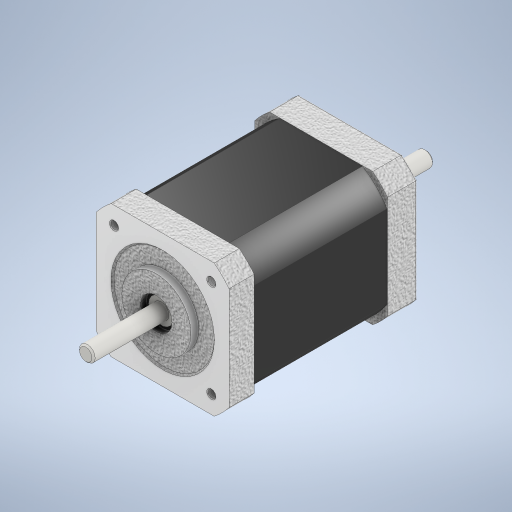
# Autodesk Inventor part: NEMA 17 Y-axis
Saved by Autodesk Inventor 2024 (Build 280153000, 153)
## iProperties
Created: 2021-02-07
Part Number: NEMA 17 Y-axis
Material: Aluminum 6061
Document SubType Name: Modeling
Designer: Ishaan
Density: 2.7 g/cm^3
Appearance: Aluminum Cast
Author: Ishaan
Autodesk Inventor part; units mm, degrees
sketch "Sketch1" plane through (0, 0, 0) normal (0, 0, 1) x (1, 0, 0)
  line L0 (21.15, -21.15) -> (-21.15, -21.15)
  line L1 (-21.15, -21.15) -> (-21.15, 21.15)
  line L2 (-21.15, 21.15) -> (21.15, 21.15)
  line L3 (21.15, 21.15) -> (21.15, -21.15)
  line L4 (21.15, -21.15) -> (-21.15, 21.15) construction
  line L5 (-21.15, -21.15) -> (21.15, 21.15) construction
  line L6 (15.5, -15.5) -> (-15.5, -15.5) construction
  line L7 (-15.5, -15.5) -> (-15.5, 15.5) construction
  line L8 (-15.5, 15.5) -> (15.5, 15.5) construction
  line L9 (15.5, 15.5) -> (15.5, -15.5) construction
  line L10 (15.5, -15.5) -> (-15.5, 15.5) construction
  line L11 (-15.5, -15.5) -> (15.5, 15.5) construction
  circle A0 centre (0, 0) radius 24.95
  circle A1 centre (0, 0) radius 11
  circle A2 centre (0, 0) radius 26.775
  point P0 (-13.2356, 21.15)
  point P1 (-21.15, 13.2356)
  point P2 (-21.15, -13.2356)
  point P3 (-13.2356, -21.15)
  point P4 (13.2356, -21.15)
  point P5 (21.15, -13.2356)
  point P6 (21.15, 13.2356)
  point P7 (13.2356, 21.15)
  point P8 (16.4188, -21.15)
  point P9 (21.15, -16.4188)
  point P10 (-21.15, -16.4188)
  point P11 (-16.4188, -21.15)
  point P12 (-16.4188, 21.15)
  point P13 (-21.15, 16.4188)
  point P14 (21.15, 16.4188)
  point P15 (16.4188, 21.15)
  dimension "d0" = 42.3
  dimension "d1" = 42.3
  dimension "d2" = 31
  dimension "d3" = 31
  dimension "d4" = 49.9
  dimension "d5" = 22
  dimension "d90" = 53.55
  constraints: 24 end point, 7 coincident, 4 midpoint, 4 parallel, 3 centre point, 2 horizontal, 2 perpendicular
  measures "d0" distance of L1.end L2.end
  measures "d1" distance of L0.end L1.end
  measures "d2" distance of L7.end L8.end
  measures "d3" distance of L6.end L7.end
  measures "d4" diameter of A0
  measures "d5" diameter of A1
  measures "d90" diameter of A2
extrude "Extrusion1" add sketch "Sketch1" against normal blind 8 contours L0 A0 L3 A2 | L0 A0 L1 L2 L3 | A2 L1 A0 L0 | A0 L2 A2 L3 | A2 L2 A0 L1 | A1
extrude "Extrusion2" add sketch "Sketch1" along normal blind 2 contours A1
hole "Hole1" at (-15.5, 15.5, 0) at (15.5, 15.5, 0) at (15.5, -15.5, 0) at (-15.5, -15.5, 0) direction (0, 0, -1) diameter 2.459 depth 4.5 thread size "M3x0.5" class "6H" standard "ANSI Metric M Profile"
ref_plane "Work Plane1" through (0, 0, -60) normal (0, 0, 1) x (1, 0, 0)
sketch "Sketch2" plane through (0, 0, -60) normal (0, 0, 1) x (1, 0, 0)
  line L0 (-16.4188, 21.15) -> (16.4188, 21.15) projected
  line L1 (21.15, 16.4188) -> (21.15, -16.4188) projected
  line L2 (16.4188, -21.15) -> (-16.4188, -21.15) projected
  line L3 (-21.15, -16.4188) -> (-21.15, 16.4188) projected
  arc A0 (-16.4188, 21.15) -> (-21.15, 16.4188) centre (0, 0) ccw projected
  arc A1 (21.15, 16.4188) -> (16.4188, 21.15) centre (0, 0) ccw projected
  arc A2 (16.4188, -21.15) -> (21.15, -16.4188) centre (0, 0) ccw projected
  arc A3 (-21.15, -16.4188) -> (-16.4188, -21.15) centre (0, 0) ccw projected
extrude "Extrusion3" add sketch "Sketch2" along normal blind 9.5
sketch "Sketch3" plane through (0, 0, -8) normal (0, 0, -1) x (-1, 0, 0)
  line L0 (16.4188, 21.15) -> (-16.4188, 21.15) projected
  line L1 (-21.15, 16.4188) -> (-21.15, -16.4188) projected
  line L2 (-16.4188, -21.15) -> (16.4188, -21.15) projected
  line L3 (21.15, -16.4188) -> (21.15, 16.4188) projected
  circle A0 centre (0, 0) radius 11 projected
  circle A1 centre (0, 0) radius 24.925
  line L4 (13.2068, -21.05) -> (-13.2068, -21.05)
  arc A2 (-21.05, -13.2068) -> (-13.2068, -21.05) centre (0, 0) ccw
  line L5 (-21.05, -13.2068) -> (-21.05, 13.2068)
  arc A3 (-13.2068, 21.05) -> (-21.05, 13.2068) centre (0, 0) ccw
  line L6 (-13.2068, 21.05) -> (13.2068, 21.05)
  arc A4 (21.05, 13.2068) -> (13.2068, 21.05) centre (0, 0) ccw
  line L7 (21.05, 13.2068) -> (21.05, -13.2068)
  arc A5 (13.2068, -21.05) -> (21.05, -13.2068) centre (0, 0) ccw
  arc A6 (21.15, 16.4188) -> (16.4188, 21.15) centre (0, 0) ccw projected
  arc A7 (-16.4188, 21.15) -> (-21.15, 16.4188) centre (0, 0) ccw projected
  arc A8 (-21.15, -16.4188) -> (-16.4188, -21.15) centre (0, 0) ccw projected
  arc A9 (16.4188, -21.15) -> (21.15, -16.4188) centre (0, 0) ccw projected
  point P0 (21.15, 13.1884)
  point P1 (13.1884, 21.15)
  point P2 (-13.1884, 21.15)
  point P3 (-21.15, 13.1884)
  point P4 (-21.15, -13.1884)
  point P5 (-13.1884, -21.15)
  point P6 (13.1884, -21.15)
  point P7 (21.15, -13.1884)
  point P8 (21.05, -13.7173)
  point P9 (21.05, 13.7173)
  point P10 (13.7173, 21.05)
  point P11 (-13.7173, 21.05)
  point P12 (-21.05, 13.7173)
  point P13 (-21.05, -13.7173)
  point P14 (-13.7173, -21.05)
  point P15 (13.7173, -21.05)
  dimension "d20" = 49.85
  dimension "d23" = 0.1
  constraints: 8 end point, 8 point on circle, 5 centre point, 1 coincident
  measures "d20" diameter of A1
  measures "d23" distance between parallel lines of L2 L4
extrude "Extrusion5" add sketch "Sketch3" along normal up to surface (42.5 mm away) contours L4 A2 L5 A3 L6 A4 L7 A5
chamfer "Chamfer1" distance 0.25 angle 45 4 edges at (-15.5, 16.7295, 0) (15.5, 16.7295, 0) (15.5, -14.2705, 0) (-15.5, -14.2705, 0)
sketch "Sketch4" plane through (0, 0, 2) normal (0, 0, 1) x (1, 0, 0)
  circle A0 centre (0, 0) radius 11 projected
  constraints: 1 coincident
hole "Hole2" at (0, 0, 2) direction (0, 0, -1) diameter 10 depth 2
sketch "Sketch5" plane through (0, 0, 0) normal (0, 0, 1) x (1, 0, 0)
  circle A0 centre (0, 0) radius 2.5
  circle A1 centre (0, 0) radius 4
  line L0 (-1.5, -2) -> (1.5, -2)
  dimension "d36" = 5
  dimension "d37" = 8
  dimension "d41" = 4.5
  constraints: 2 centre point, 2 coincident, 2 end point, 2 point on circle, 1 horizontal
  measures "d36" diameter of A0
  measures "d37" diameter of A1
ref_plane "Work Plane2" through (0, 0, 24.5) normal (0, 0, 1) x (1, 0, 0)
extrude "Extrusion6" add sketch "Sketch5" along normal up to surface (24.5 mm away) contours A0 L0 | L0 A0
chamfer "Chamfer2" distance 0.5 angle 45 1 edges at (1.5, 2, 24.5)
extrude "Extrusion7" cut sketch "Sketch5" along normal blind 22.298 from surface at 2 contours L0 A0 picked at (-0.3466, -2.0912)
extrude "Extrusion8" add sketch "Sketch5" along normal blind 0.5
sketch "Sketch6" plane through (0, 0, -60) normal (0, 0, -1) x (-1, 0, 0)
  circle A0 centre (0, 0) radius 5
  dimension "d49" = 10
  constraints: 1 centre point, 1 coincident
  measures "d49" diameter of A0
extrude "Extrusion9" cut sketch "Sketch6" against normal blind 3
sketch "Sketch7" plane through (0, 0, -57) normal (0, 0, -1) x (-1, 0, 0)
  circle A0 centre (0, 0) radius 4
  circle A1 centre (0, 0) radius 2.5
  dimension "d52" = 8
  dimension "d53" = 5
  constraints: 2 centre point, 2 coincident
  measures "d52" diameter of A0
  measures "d53" diameter of A1
ref_plane "Work Plane4" through (0, 0, -84) normal (0, 0, -1) x (-1, 0, 0)
extrude "Extrusion10" add sketch "Sketch7" along normal up to surface (27 mm away) contours A1
ref_plane "Work Plane5" through (0, 0, -69) normal (0, 0, -1) x (-1, 0, 0)
chamfer "Chamfer5" distance 0.5 angle 45 1 edges at (2.5, 0, -84)
sketch "Sketch11" plane through (0, 0, -69) normal (0, 0, -1) x (-1, 0, 0)
  circle A0 centre (0, 0) radius 2.5 projected
  line L0 (1.5, -2) -> (-1.5, -2)
  dimension "d94" = 2
  constraints: 2 end point, 2 point on circle, 1 horizontal
  measures "d94" distance from line of L0 point (0, 0)
extrude "Extrusion15" cut sketch "Sketch11" along normal through all contours L0 A0 picked at (-0.3466, -2.0912)
extrude "Extrusion11" add sketch "Sketch7" along normal blind 0.5
sketch "Sketch8" plane through (0, 0, -60) normal (0, 0, -1) x (-1, 0, 0)
  circle A0 centre (-15.5, 15.5) radius 1.2295 projected
  circle A1 centre (-15.5, 15.5) radius 3.25
  circle A2 centre (15.5, 15.5) radius 1.2295 projected
  circle A3 centre (15.5, 15.5) radius 3.25
  circle A4 centre (15.5, -15.5) radius 3.25
  circle A5 centre (-15.5, -15.5) radius 1.2295 projected
  circle A6 centre (-15.5, -15.5) radius 3.25
  line L0 (12.25, -21.15) -> (-12.25, -21.15)
  line L1 (-12.25, -21.15) -> (-12.25, 21.15)
  line L2 (-12.25, 21.15) -> (12.25, 21.15)
  line L3 (12.25, 21.15) -> (12.25, -21.15)
  circle A7 centre (0, 0) radius 4 projected
  line L4 (12.25, -21.15) -> (-12.25, 21.15) construction
  line L5 (-12.25, -21.15) -> (12.25, 21.15) construction
  line L6 (21.15, -12.25) -> (-21.15, -12.25)
  line L7 (-21.15, -12.25) -> (-21.15, 12.25)
  line L8 (-21.15, 12.25) -> (21.15, 12.25)
  line L9 (21.15, 12.25) -> (21.15, -12.25)
  line L10 (21.15, -12.25) -> (-21.15, 12.25) construction
  line L11 (-21.15, -12.25) -> (21.15, 12.25) construction
  line L12 (-16.4188, 21.15) -> (16.4188, 21.15) projected
  line L13 (21.15, 16.4188) -> (21.15, -16.4188) projected
  circle A8 centre (0, 0) radius 5 projected
  line L14 (16.4188, -21.15) -> (-16.4188, -21.15) projected
  line L15 (21.15, 16.4188) -> (21.15, -16.4188) projected
  line L16 (-16.4188, 21.15) -> (16.4188, 21.15) projected
  line L17 (-21.15, -16.4188) -> (-21.15, 16.4188) projected
  arc A9 (-16.4188, 21.15) -> (-21.15, 16.4188) centre (0, 0) ccw projected
  arc A10 (-21.15, -16.4188) -> (-16.4188, -21.15) centre (0, 0) ccw projected
  arc A11 (16.4188, -21.15) -> (21.15, -16.4188) centre (0, 0) ccw projected
  arc A12 (21.15, 16.4188) -> (16.4188, 21.15) centre (0, 0) ccw projected
  point P0 (-13.2356, 21.15)
  point P1 (13.2356, 21.15)
  point P2 (21.15, 13.2356)
  point P3 (21.15, -13.2356)
  point P4 (12.25, 21.15)
  point P5 (12.25, 15.5)
  point P6 (15.5, 12.25)
  point P7 (12.25, -12.25)
  point P8 (12.25, 12.25)
  point P9 (-12.25, 12.25)
  point P10 (-12.25, -12.25)
  point P11 (-12.25, -21.15)
  dimension "d72" = 24.5
  constraints: 24 end point, 4 centre point, 4 coincident, 4 midpoint, 4 parallel, 3 equal radius, 2 horizontal, 2 perpendicular, 2 point on line, 2 tangent
  measures "d72" distance between parallel lines of L8 L6
extrude "Extrusion13" cut sketch "Sketch8" against normal blind 2 contours A0 | A1 | A3 | A6 | A4 | A2 | A5
fillet "Fillet3" radius 0.5 12 edges at (21.15, 0, -60) (18.75, -15.5, -60) (0, -21.15, -60) (-12.25, -15.5, -60) (-21.15, 0, -60) (0, 21.15, -60) (18.9328, -18.9328, -60) (-18.9328, -18.9328, -60) (-18.9328, 18.9328, -60) (18.9328, 18.9328, -60) (-12.25, 15.5, -60) (18.75, 15.5, -60)
sketch "Sketch9" plane through (-15.5, -15.5, -58) normal (0, 0, -1) x (-1, 0, 0)
  circle A0 centre (0, 0) radius 3 projected
  line L0 (-36.65, -0.9188) -> (-36.65, 31.9188) projected
  line L1 (-3.25, 27.75) -> (-27.75, 27.75) projected
  line L2 (-31.9188, 36.65) -> (0.9188, 36.65) projected
  circle A1 centre (-31, 31) radius 2.75
  line L3 (-3.25, 3.25) -> (-3.25, 27.75) projected
  line L4 (-27.75, 3.25) -> (-3.25, 3.25) projected
  line L5 (-27.75, 27.75) -> (-27.75, 3.25) projected
  line L6 (5.65, 31.9188) -> (5.65, -0.9188) projected
  arc A2 (5.65, 31.9188) -> (0.9188, 36.65) centre (-15.5, 15.5) ccw projected
  arc A3 (-31.9188, 36.65) -> (-36.65, 31.9188) centre (-15.5, 15.5) ccw projected
  arc A4 (-36.65, -0.9188) -> (-31.9188, -5.65) centre (-15.5, 15.5) ccw projected
  line L7 (0.9188, -5.65) -> (-31.9188, -5.65) projected
  arc A5 (0.9188, -5.65) -> (5.65, -0.9188) centre (-15.5, 15.5) ccw projected
  dimension "d80" = 5.5
  constraints: 1 centre point
  measures "d80" diameter of A1
extrude "Extrusion12" add sketch "Sketch9" along normal blind 2 contours A1
fillet "Fillet1" radius 0.5 1 edges at (18.25, 15.5, -60)
pattern_circular "Circular Pattern2" count 4 over 360 about axis through (0, 0, -60) along (0, 0, 1) of "Extrusion12", "Fillet1"
sketch "Sketch10" plane through (0, 0, 0) normal (0, 0, 1) x (1, 0, 0)
  circle A0 centre (15.5, -15.5) radius 1.4795 projected
  circle A1 centre (-15.5, 15.5) radius 1.4795 projected
  circle A2 centre (0, 0) radius 11 projected
  line L0 (16.4188, 21.15) -> (-16.4188, 21.15) projected
  line L1 (-21.15, 16.4188) -> (-21.15, -16.4188) projected
  line L2 (-16.4188, -21.15) -> (16.4188, -21.15) projected
  line L3 (21.15, -16.4188) -> (21.15, 16.4188) projected
  circle A3 centre (15.5, 15.5) radius 1.4795 projected
  circle A4 centre (-15.5, -15.5) radius 1.4795 projected
  circle A5 centre (0, 0) radius 16
  arc A6 (-21.15, -16.4188) -> (-16.4188, -21.15) centre (0, 0) ccw projected
  arc A7 (16.4188, -21.15) -> (21.15, -16.4188) centre (0, 0) ccw projected
  arc A8 (21.15, 16.4188) -> (16.4188, 21.15) centre (0, 0) ccw projected
  arc A9 (-16.4188, 21.15) -> (-21.15, 16.4188) centre (0, 0) ccw projected
  dimension "d84" = 32
  constraints: 1 centre point
  measures "d84" diameter of A5
extrude "Extrusion14" cut sketch "Sketch10" against normal blind 0.5 contours A5
chamfer "Chamfer4" distance 0.5 angle 45 1 edges at (-16, 0, 0)
body "Solid1"
